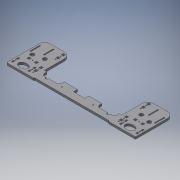
# Autodesk Inventor part: A8-0010
Saved by Autodesk Inventor 2016 SP2 (Build 200236200, 236)
## iProperties
Created: 2017-04-22
Part Number: A8-0010
Material: Generic
Document SubType Name: Modeling
Designer: EV
Density: 1 g/cm^3
Appearance: Default
Author: EV
Autodesk Inventor part; units mm, degrees
ref_plane "YZ Plane" through (0, 0, 0) normal (1, 0, 0) x (0, 1, 0)
ref_plane "XZ Plane" through (0, 0, 0) normal (0, 1, 0) x (-1, 0, 0)
ref_plane "XY Plane" through (0, 0, 0) normal (0, 0, 1) x (1, 0, 0)
sketch "Sketch1" plane through (0, 0, 0) normal (0, 1, 0) x (-1, 0, 0)
  line L0 (-227.75, 0) -> (-133.75, 0)
  line L1 (-133.75, 0) -> (-130.75, -3)
  line L2 (-130.75, -3) -> (130.75, -3)
  line L3 (130.75, -3) -> (133.75, 0)
  line L4 (133.75, 0) -> (227.75, 0)
  line L5 (227.75, 0) -> (227.75, -114)
  line L6 (207.75, -134) -> (157.25, -134)
  line L7 (137.25, -114) -> (137.25, -42.5)
  line L8 (137.25, -42.5) -> (128.25, -42.5)
  line L9 (128.25, -42.5) -> (128.25, -34.5)
  line L10 (66.25, -34.5) -> (66.25, -42.5)
  line L11 (66.25, -42.5) -> (20.25, -42.5)
  line L12 (20.25, -42.5) -> (20.25, -28.5)
  line L13 (20.25, -28.5) -> (-20.25, -28.5)
  line L14 (-20.25, -28.5) -> (-20.25, -42.5)
  line L15 (-20.25, -42.5) -> (-66.25, -42.5)
  line L16 (-66.25, -42.5) -> (-66.25, -34.5)
  line L17 (-128.25, -34.5) -> (-128.25, -42.5)
  line L18 (-128.25, -42.5) -> (-137.25, -42.5)
  line L19 (-137.25, -42.5) -> (-137.25, -114)
  line L20 (-157.25, -134) -> (-207.75, -134)
  line L21 (-227.75, -114) -> (-227.75, 0)
  line L22 (0, -3) -> (0, 0) construction
  line L23 (0, -3) -> (0, -28.5) construction
  arc A0 (207.75, -134) -> (227.75, -114) centre (207.75, -114) ccw
  arc A1 (137.25, -114) -> (157.25, -134) centre (157.25, -114) ccw
  arc A2 (-157.25, -134) -> (-137.25, -114) centre (-157.25, -114) ccw
  arc A3 (-227.75, -114) -> (-207.75, -134) centre (-207.75, -114) ccw
  arc A4 (128.25, -34.5) -> (118.25, -24.5) centre (118.25, -34.5) ccw
  arc A5 (76.25, -24.5) -> (66.25, -34.5) centre (76.25, -34.5) ccw
  arc A6 (-66.25, -34.5) -> (-76.25, -24.5) centre (-76.25, -34.5) ccw
  arc A7 (-118.25, -24.5) -> (-128.25, -34.5) centre (-118.25, -34.5) ccw
  line L24 (108.75, -24.5) -> (108.75, -22.75) construction
  line L25 (113, -24.5) -> (113, -22.75)
  line L26 (104.5, -22.75) -> (104.5, -24.5)
  arc A8 (113, -22.75) -> (104.5, -22.75) centre (108.75, -22.75) ccw
  line L27 (-108.75, -24.5) -> (-108.75, -22.75) construction
  line L28 (-104.5, -24.5) -> (-104.5, -22.75)
  line L29 (-113, -22.75) -> (-113, -24.5)
  arc A9 (-104.5, -22.75) -> (-113, -22.75) centre (-108.75, -22.75) ccw
  line L30 (-76.25, -24.5) -> (-104.5, -24.5)
  line L31 (-113, -24.5) -> (-118.25, -24.5)
  line L32 (118.25, -24.5) -> (113, -24.5)
  line L33 (104.5, -24.5) -> (76.25, -24.5)
  dimension "d0" = 455.5
  dimension "d1" = 45
  dimension "d2" = 3
  dimension "d3" = 94
  dimension "d4" = 134
  dimension "d5" = 25.5
  dimension "d6" = 39.5
  dimension "d8" = 40.5
  dimension "d9" = 46
  dimension "d11" = 90.5
  dimension "d12" = 20
  dimension "d13" = 10
  dimension "d14" = 21.5
  dimension "d15" = 8.5
  dimension "d17" = 119
  dimension "d18" = 15.5
  dimension "d19" = 62
  constraints: 71 end point, 24 tangent, 20 perpendicular, 20 point on circle, 11 point on line, 10 centre point, 10 collinear, 7 equal radius, 5 vertical, 3 parallel, 2 midpoint, 1 horizontal, 1 vertical alignment, 1 other
  measures "d0" distance between parallel lines of L21 L5
  measures "d1" angle of L3 L4
  measures "d2" distance from line of L22.end L2
  measures "d3" distance of L3.end L4.end
  measures "d4" distance between parallel lines of L6 L4
  measures "d5" distance between parallel lines of L2 L13
  measures "d6" distance between parallel lines of L11 L2
  measures "d8" distance of L12.end L13.end
  measures "d9" distance of L10.end L11.end
  measures "d11" distance between parallel lines of L5 L7
  measures "d12" radius of A0
  measures "d13" radius of A4
  measures "d14" distance between parallel lines of L2 L33
  measures "d15" distance between parallel lines of L25 L26
  measures "d17" distance between parallel lines of L5 L24
  measures "d18" distance edge to line of A8 L2
  measures "d19" distance between parallel lines of L10 L9
extrude "Extrusion1" add sketch "Sketch1" along normal blind 8
sketch "Sketch2" plane through (0, 8, 0) normal (0, 1, 0) x (1, 0, 0)
  line L0 (133.75, 0) -> (227.75, 0) construction
  line L1 (227.75, 0) -> (227.75, 114) construction
  arc A0 (227.75, 114) -> (207.75, 134) centre (207.75, 114) ccw construction
  line L2 (207.75, 134) -> (157.25, 134) construction
  arc A1 (157.25, 134) -> (137.25, 114) centre (157.25, 114) ccw construction
  line L3 (137.25, 114) -> (137.25, 42.5) construction
  line L4 (137.25, 42.5) -> (128.25, 42.5) construction
  line L5 (128.25, 42.5) -> (128.25, 34.5) construction
  arc A2 (118.25, 24.5) -> (128.25, 34.5) centre (118.25, 34.5) ccw construction
  line L6 (118.25, 24.5) -> (113, 24.5) construction
  line L7 (113, 24.5) -> (113, 22.75) construction
  arc A3 (104.5, 22.75) -> (113, 22.75) centre (108.75, 22.75) ccw construction
  line L8 (104.5, 22.75) -> (104.5, 24.5) construction
  line L9 (104.5, 24.5) -> (76.25, 24.5) construction
  arc A4 (66.25, 34.5) -> (76.25, 24.5) centre (76.25, 34.5) ccw construction
  line L10 (66.25, 34.5) -> (66.25, 42.5) construction
  line L11 (66.25, 42.5) -> (20.25, 42.5) construction
  line L12 (20.25, 42.5) -> (20.25, 28.5) construction
  line L13 (20.25, 28.5) -> (-20.25, 28.5) construction
  line L14 (-20.25, 28.5) -> (-20.25, 42.5) construction
  line L15 (-20.25, 42.5) -> (-66.25, 42.5) construction
  line L16 (-66.25, 42.5) -> (-66.25, 34.5) construction
  arc A5 (-76.25, 24.5) -> (-66.25, 34.5) centre (-76.25, 34.5) ccw construction
  line L17 (-76.25, 24.5) -> (-104.5, 24.5) construction
  line L18 (-104.5, 24.5) -> (-104.5, 22.75) construction
  arc A6 (-113, 22.75) -> (-104.5, 22.75) centre (-108.75, 22.75) ccw construction
  line L19 (-113, 22.75) -> (-113, 24.5) construction
  line L20 (-113, 24.5) -> (-118.25, 24.5) construction
  arc A7 (-128.25, 34.5) -> (-118.25, 24.5) centre (-118.25, 34.5) ccw construction
  line L21 (-128.25, 34.5) -> (-128.25, 42.5) construction
  line L22 (-128.25, 42.5) -> (-137.25, 42.5) construction
  line L23 (-137.25, 42.5) -> (-137.25, 114) construction
  arc A8 (-137.25, 114) -> (-157.25, 134) centre (-157.25, 114) ccw construction
  line L24 (-157.25, 134) -> (-207.75, 134) construction
  arc A9 (-207.75, 134) -> (-227.75, 114) centre (-207.75, 114) ccw construction
  line L25 (-227.75, 114) -> (-227.75, 0) construction
  line L26 (-227.75, 0) -> (-133.75, 0) construction
  line L27 (-133.75, 0) -> (-130.75, 3) construction
  line L28 (-130.75, 3) -> (130.75, 3) construction
  line L29 (130.75, 3) -> (133.75, 0) construction
  line L30 (-220.25, 111.5) -> (-220.25, 75) construction
  line L31 (-222.25, 109.5) -> (-222.25, 77)
  line L32 (-218.25, 77) -> (-218.25, 109.5)
  arc A10 (-218.25, 109.5) -> (-222.25, 109.5) centre (-220.25, 109.5) ccw
  arc A11 (-222.25, 77) -> (-218.25, 77) centre (-220.25, 77) ccw
  line L33 (-185.25, 124.5) -> (-185.25, 88) construction
  line L34 (-187.25, 122.5) -> (-187.25, 90)
  line L35 (-183.25, 90) -> (-183.25, 122.5)
  arc A12 (-183.25, 122.5) -> (-187.25, 122.5) centre (-185.25, 122.5) ccw
  arc A13 (-187.25, 90) -> (-183.25, 90) centre (-185.25, 90) ccw
  line L36 (-222.5, 28.7) -> (-217, 28.7)
  line L37 (-217, 28.7) -> (-217, 36.9)
  line L38 (-217, 36.9) -> (-222.5, 36.9)
  line L39 (-222.5, 36.9) -> (-222.5, 28.7)
  line L40 (-222.5, 19.2) -> (-217, 19.2)
  line L41 (-217, 19.2) -> (-217, 11)
  line L42 (-217, 11) -> (-222.5, 11)
  line L43 (-222.5, 11) -> (-222.5, 19.2)
  line L44 (-205.25, 56.95) -> (-197.05, 56.95)
  line L45 (-197.05, 56.95) -> (-197.05, 48.75)
  line L46 (-197.05, 48.75) -> (-205.25, 48.75)
  line L47 (-205.25, 48.75) -> (-205.25, 56.95)
  line L48 (-179.55, 56.95) -> (-171.35, 56.95)
  line L49 (-171.35, 56.95) -> (-171.35, 48.75)
  line L50 (-171.35, 48.75) -> (-179.55, 48.75)
  line L51 (-179.55, 48.75) -> (-179.55, 56.95)
  line L52 (-164.5, 36.9) -> (-159, 36.9)
  line L53 (-159, 36.9) -> (-159, 28.7)
  line L54 (-159, 28.7) -> (-164.5, 28.7)
  line L55 (-164.5, 28.7) -> (-164.5, 36.9)
  line L56 (-164.5, 19.2) -> (-159, 19.2)
  line L57 (-159, 19.2) -> (-159, 11)
  line L58 (-159, 11) -> (-164.5, 11)
  line L59 (-164.5, 11) -> (-164.5, 19.2)
  line L60 (-155.25, 49.4) -> (-147.05, 49.4)
  line L61 (-147.05, 49.4) -> (-147.05, 41.2)
  line L62 (-147.05, 41.2) -> (-155.25, 41.2)
  line L63 (-155.25, 41.2) -> (-155.25, 49.4)
  line L64 (-155.25, 30.7) -> (-147.05, 30.7)
  line L65 (-147.05, 30.7) -> (-147.05, 22.5)
  line L66 (-147.05, 22.5) -> (-155.25, 22.5)
  line L67 (-155.25, 22.5) -> (-155.25, 30.7)
  line L68 (-155.25, 127.9) -> (-147.05, 127.9)
  line L69 (-147.05, 127.9) -> (-147.05, 119.7)
  line L70 (-147.05, 119.7) -> (-155.25, 119.7)
  line L71 (-155.25, 119.7) -> (-155.25, 127.9)
  line L72 (-155.25, 109.2) -> (-147.05, 109.2)
  line L73 (-147.05, 109.2) -> (-147.05, 101)
  line L74 (-147.05, 101) -> (-155.25, 101)
  line L75 (-155.25, 101) -> (-155.25, 109.2)
  line L76 (-219.75, 11) -> (-219.75, 36.9) construction
  line L77 (-205.25, 52.85) -> (-171.35, 52.85) construction
  line L78 (-161.75, 36.9) -> (-161.75, 11) construction
  line L79 (-151.15, 22.5) -> (-151.15, 49.4) construction
  line L80 (-151.15, 127.9) -> (-151.15, 101) construction
  ellipse E0 centre (-188.75, 20) end of major axis (-171.25, 20) minor radius 12.5
  point P0 (0, 0)
  point P1 (-220.25, 93.25)
  point P2 (-185.25, 106.25)
  point P3 (-219.75, 23.95)
  point P4 (-188.3, 52.85)
  point P5 (-161.75, 23.95)
  point P6 (-151.15, 35.95)
  point P7 (-151.15, 17.5)
  point P8 (-151.15, 114.45)
  point P9 (-151.15, 96)
  point P10 (-55.25, 23)
  point P11 (-206.75, 69.5)
  point P12 (-170.75, 78)
  dimension "d62" = 17.5
  dimension "d63" = 12.5
  dimension "d22" = 7.5
  dimension "d23" = 42.5
  dimension "d24" = 36.5
  dimension "d25" = 36.5
  dimension "d26" = 4
  dimension "d27" = 4
  dimension "d28" = 75
  dimension "d29" = 88
  dimension "d30" = 5.5
  dimension "d31" = 8.2
  dimension "d32" = 5.5
  dimension "d33" = 8.2
  dimension "d34" = 8.2
  dimension "d35" = 8.2
  dimension "d36" = 8.2
  dimension "d37" = 8.2
  dimension "d38" = 8.2
  dimension "d39" = 8.2
  dimension "d40" = 9.5
  dimension "d41" = 17.5
  dimension "d42" = 9.5
  dimension "d43" = 10.5
  dimension "d44" = 10.5
  dimension "d46" = 5.25
  dimension "d47" = 22.5
  dimension "d48" = 63.25
  dimension "d49" = 72.5
  dimension "d50" = 72.5
  dimension "d51" = 11
  dimension "d52" = 11
  dimension "d53" = 48.75
  dimension "d54" = 22.5
  dimension "d55" = 101
  dimension "d56" = 5
  dimension "d57" = 5
  dimension "d58" = 20
  dimension "d59" = 11
  dimension "d60" = 20
  dimension "d61" = 39
  dimension "d64" = 21
  dimension "d65" = 57
  dimension "d66" = 69.5
  dimension "d67" = 78
  constraints: 106 end point, 22 parallel, 17 midpoint, 12 point on circle, 11 horizontal, 10 equal length, 10 perpendicular, 8 tangent, 6 point on line, 6 vertical, 4 centre point, 2 other
  measures "d22" distance between parallel lines of L25 L30
  measures "d23" distance between parallel lines of L25 L33
  measures "d24" distance of L30.start L30.end
  measures "d25" distance of L33.start L33.end
  measures "d26" distance between parallel lines of L32 L31
  measures "d27" distance between parallel lines of L35 L34
  measures "d28" distance from line of L26 L30.end
  measures "d29" distance from line of L26 L33.end
  measures "d30" distance of L41.end L42.end
  measures "d31" distance of L45.end L46.end
  measures "d32" distance of L57.end L58.end
  measures "d33" distance of L65.end L66.end
  measures "d34" distance of L73.end L74.end
  measures "d35" distance of L42.end L40.start
  measures "d36" distance of L46.end L44.start
  measures "d37" distance of L58.end L56.start
  measures "d38" distance of L66.end L64.start
  measures "d39" distance of L74.end L72.start
  measures "d40" distance between parallel lines of L36 L40
  measures "d41" distance between parallel lines of L51 L45
  measures "d42" distance between parallel lines of L56 L54
  measures "d43" distance between parallel lines of L62 L64
  measures "d44" distance between parallel lines of L70 L72
  measures "d46" distance between parallel lines of L25 L43
  measures "d47" distance between parallel lines of L25 L47
  measures "d48" distance between parallel lines of L25 L59
  measures "d49" distance between parallel lines of L25 L67
  measures "d50" distance between parallel lines of L25 L75
  measures "d51" distance between parallel lines of L42 L26
  measures "d52" distance between parallel lines of L26 L58
  measures "d53" distance between parallel lines of L26 L46
  measures "d54" distance between parallel lines of L26 L66
  measures "d55" distance between parallel lines of L74 L26
  measures "d56" distance from line of L66 point (-151.15, 17.5)
  measures "d57" distance from line of L74 point (-151.15, 96)
  measures "d58" distance from line of L28 point (-55.25, 23)
  measures "d59" distance from line of L16 point (-55.25, 23)
  measures "d60" distance from line of L26 point (-188.75, 20)
  measures "d61" distance from line of L25 point (-188.75, 20)
  measures "d64" distance from line of L25 point (-206.75, 69.5)
  measures "d65" distance from line of L25 point (-170.75, 78)
  measures "d66" distance from line of point (-206.75, 69.5) L26
  measures "d67" distance from line of L26 point (-170.75, 78)
extrude "Extrusion2" cut sketch "Sketch2" against normal through all
hole "Hole1" at (-219.75, 8, -23.95) at (-188.3, 8, -52.85) at (-161.75, 8, -23.95) at (-151.15, 8, -35.95) at (-151.15, 8, -17.5) at (-151.15, 8, -114.45) at (-151.15, 8, -96) at (-55.25, 8, -23) direction (0, -1, 0) diameter 3.5 end through all
hole "Hole2" at (-206.75, 8, -69.5) at (-170.75, 8, -78) direction (0, -1, 0) diameter 14 end through all
mirror "Mirror1" about plane through (0, 0, 0) normal (1, 0, 0) of "Extrusion2", "Hole1", "Hole2"
fillet "Fillet1" radius 2 6 edges at (-133.75, 4, 0) (-130.75, 4, -3) (130.75, 4, -3) (133.75, 4, 0) (227.75, 4, 0) (-227.75, 4, 0)
equation "\"d25\" = d24"
equation "\"d27\" = d26"
body "Solid1"
